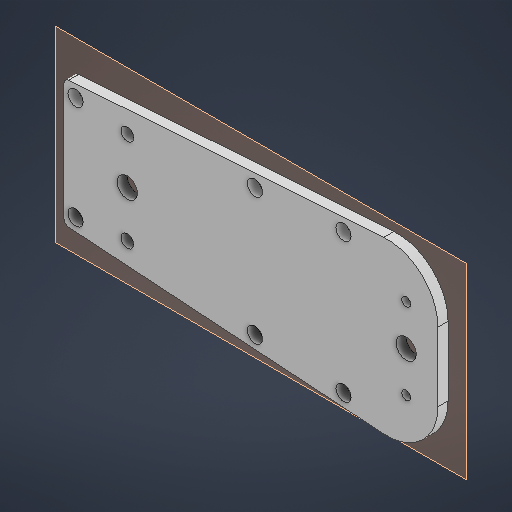
# Autodesk Inventor part: El0-2
Saved by Autodesk Inventor 2025.3 (Build 293356000, 356)
## iProperties
Created: 2025-04-19
Part Number: El0-2
Material: Generic
Document SubType Name: Modeling
Designer: Nelson
Density: 1 g/cm^3
Appearance: Default
Author: Nelson
Autodesk Inventor part; units mm, degrees
ref_plane "YZ Plane" through (0, 0, 0) normal (1, 0, 0) x (0, 1, 0)
ref_plane "XZ Plane" through (0, 0, 0) normal (0, 1, 0) x (-1, 0, 0)
sketch "Sketch1" plane through (0, 0, 0) normal (0, 0, 1) x (1, 0, 0)
  line L0 (-60, 0) -> (60, 0)
  line L1 (-35, -25) -> (-85, -25)
  line L2 (-85, -25) -> (-85, 25)
  line L3 (-85, 25) -> (-35, 25)
  line L4 (-35, 25) -> (-35, -25) construction
  line L5 (-35, -25) -> (-85, 25) construction
  line L6 (-85, -25) -> (-35, 25) construction
  circle A0 centre (-60, 0) radius 24.373 construction
  line L7 (62.5, -35) -> (17.5, -35)
  line L8 (17.5, -35) -> (17.5, 35) construction
  line L9 (17.5, 35) -> (62.5, 35)
  line L10 (62.5, 35) -> (62.5, -35)
  line L11 (62.5, -35) -> (17.5, 35) construction
  line L12 (17.5, -35) -> (62.5, 35) construction
  line L13 (62.5, 35) -> (-85, 25)
  line L14 (62.5, -35) -> (-85, -25)
  line L15 (-60, 0) -> (99.4625, 0)
  line L16 (78.3125, -21.15) -> (120.6125, -21.15) construction
  line L17 (120.6125, -21.15) -> (120.6125, 21.15) construction
  line L18 (120.6125, 21.15) -> (78.3125, 21.15) construction
  line L19 (78.3125, 21.15) -> (78.3125, -21.15) construction
  line L20 (78.3125, -21.15) -> (120.6125, 21.15) construction
  line L21 (120.6125, -21.15) -> (78.3125, 21.15) construction
  circle A1 centre (50, 0) radius 37.5 construction
  circle A2 centre (99.4625, 0) radius 9 construction
  circle A3 centre (50, 0) radius 4
  line L22 (-85, -25) -> (-80.4038, -20.4038)
  circle A4 centre (-80.4038, -20.4038) radius 3
  line L23 (-10, -30.0847) -> (-9.6618, -25.0962)
  circle A5 centre (-9.6618, -25.0962) radius 3
  circle A6 centre (-80.4038, 20.4038) radius 3
  circle A7 centre (-9.6618, 25.0962) radius 3
  line L24 (50, 0) -> (50, 16)
  circle A8 centre (50, 16) radius 1.75
  circle A9 centre (50, -16) radius 1.75
  circle A10 centre (50, 0) radius 10 construction
  line L25 (-9.6618, -25.0962) -> (25.258, -27.4636) construction
  circle A11 centre (25.258, -27.4636) radius 3
  circle A12 centre (25.258, 27.4636) radius 3
  circle A13 centre (99.4625, 0) radius 2.5
  circle A14 centre (99.4625, 0) radius 11
  line L26 (-60, 0) -> (-60, 18.25)
  circle A15 centre (-60, 18.25) radius 2.5
  circle A16 centre (-60, -18.25) radius 2.5
  circle A17 centre (-60, 0) radius 4
  point P0 (0, 0)
  dimension "d0" = 120
  dimension "d1" = 50
  dimension "d2" = 50
  dimension "d3" = 48.746
  dimension "d5" = 45
  dimension "d6" = 70
  dimension "d9" = 159.4625
  dimension "d10" = 42.3
  dimension "d11" = 42.3
  dimension "d12" = 75
  dimension "d14" = 18
  dimension "d15" = 8
  dimension "d16" = 6.5
  dimension "d17" = 6
  dimension "d18" = 5
  dimension "d19" = 6
  dimension "d25" = 16
  dimension "d26" = 3.5
  dimension "d27" = 20
  dimension "d28" = 35
  dimension "D" = 6
  dimension "d31" = 5
  dimension "d32" = 22
  dimension "d33" = 18.25
  dimension "d34" = 5
  dimension "d35" = 8
  constraints: 54 end point, 18 centre point, 12 coincident, 7 parallel, 5 midpoint, 5 perpendicular, 5 symmetric about line, 4 horizontal, 3 point on line, 1 vertical, 5 other
  measures "d0" distance of L0.start L0.end
  measures "d1" distance of L2.end L3.end
  measures "d2" distance of L1.end L2.end
  measures "d3" diameter of A0
  measures "d5" distance of L8.end L9.end
  measures "d6" distance of L9.end L7.start
  measures "d9" distance of L15.start L15.end
  measures "d10" distance of L18.end L17.end
  measures "d11" distance of L16.end L17.end
  measures "d12" diameter of A1
  measures "d14" diameter of A2
  measures "d15" diameter of A3
  measures "d16" distance of L1.end L22.end
  measures "d17" diameter of A4
  measures "d18" distance of L23.start L23.end
  measures "d19" diameter of A5
  measures "d25" distance of L24.start L24.end
  measures "d26" diameter of A8
  measures "d27" diameter of A10
  measures "d28" distance of L25.start L25.end
  measures "D" diameter of A11
  measures "d31" diameter of A13
  measures "d32" diameter of A14
  measures "d33" distance of L15.start L26.end
  measures "d34" diameter of A15
  measures "d35" diameter of A17
extrude "Extrusion1" add sketch "Sketch1" along normal blind 4 contours L2 L13 L10 L14
fillet "Fillet1" radius 2 2 edges at (-85, -25, 2) (-85, 25, 2)
fillet "Fillet3" radius 20 2 edges at (62.5, -35, 2) (62.5, 35, 2)
equation "\"d17\" = D"
equation "\"d19\" = D"
body "Solid1"
